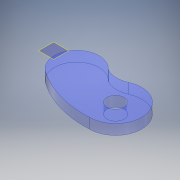
# Autodesk Inventor part: body depart
Saved by Autodesk Inventor 2018.1 (Build 221171000, 171)
## iProperties
Created: 2022-07-20
Part Number: body depart
Material: Generic
Document SubType Name: Modeling
Designer: mouta
Density: 1 g/cm^3
Appearance: Default
Author: mouta
Autodesk Inventor part; units mm, degrees
ref_plane "YZ Plane" through (0, 0, 0) normal (1, 0, 0) x (0, 1, 0)
ref_plane "XZ Plane" through (0, 0, 0) normal (0, 1, 0) x (-1, 0, 0)
ref_plane "XY Plane" through (0, 0, 0) normal (0, 0, 1) x (1, 0, 0)
ref_plane "Work Plane1" through (0, 0, 0) normal (0, 0, -1) x (-1, 0, 0)
sketch "Sketch2" plane through (0, 0, 0) normal (0, 0, -1) x (-1, 0, 0)
  circle A0 centre (-110.2989, -19.8991) radius 12.5 projected
  arc A1 (-94.6273, 14.7187) -> (-110.2989, -57.8991) centre (-110.2989, -19.8991) ccw
  arc A2 (-20.6621, -32.3715) -> (-63.0975, 16.6001) centre (-39.2432, -5.6011) ccw
  arc A3 (-94.6273, 14.7187) -> (-64.4404, 15.5759) centre (-80.4132, 46.1169) ccw
  arc A4 (-110.2989, -57.8991) -> (-20.6621, -32.3715) centre (-102.829, 86.0087) ccw
  arc A5 (-64.4404, 15.5759) -> (-63.0975, 16.6001) centre (-66.7576, 20.0065) ccw
  point P0 (0, 0)
  dimension "d38" = 76
  dimension "d39" = 5
  constraints: 10 point on circle, 5 centre point, 4 tangent, 1 coincident
  measures "d38" diameter of A1
  measures "d39" radius of A5
extrude "Extrusion4" add sketch "Sketch2" along normal blind 15
body "Solid3"
